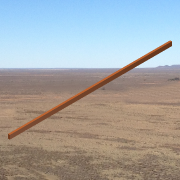
# Autodesk Inventor part: 2p4rim
Saved by Autodesk Inventor 2014 SP1 (Build 180222100, 222)
## iProperties
Company: HERA Project
Created: 2013-12-03
Part Number: 2p4rim
Material: Wood (Cherry)
Document SubType Name: Modeling
Designer: David DeBoer
Mass: 5807.17 g
Surface Area: 8777.4 cm^2
Volume: 11614.3 cm^3
Density: 0.5 g/cm^3
Description: rim piece
Appearance: Cherry - Natural Low Gloss
Author: David DeBoer
Autodesk Inventor part; units mm, degrees
ref_plane "YZ Plane" through (0, 0, 0) normal (1, 0, 0) x (0, 1, 0)
ref_plane "XZ Plane" through (0, 0, 0) normal (0, 1, 0) x (-1, 0, 0)
ref_plane "XY Plane" through (0, 0, 0) normal (0, 0, 1) x (1, 0, 0)
sketch "Sketch1" plane through (0, 0, 0) normal (0, 0, 1) x (1, 0, 0)
  line L0 (0, 0) -> (38.1, 0)
  line L1 (38.1, 0) -> (38.1, 88.9)
  line L2 (38.1, 88.9) -> (0, 88.9)
  line L3 (0, 88.9) -> (0, 0)
  dimension "d0" = 38.1
  dimension "d1" = 88.9
  constraints: 8 end point, 2 parallel, 1 horizontal, 1 perpendicular
  measures "d0" distance of L0.start L0.end
  measures "d1" distance of L2.end L0.start
extrude "Extrusion1" add sketch "Sketch1" along normal blind 3502.025
sketch "Sketch2" plane through (38.1, 0, 0) normal (0, -1, 0) x (1, 0, 0)
  line L0 (0, 0) -> (0, 3502.025) projected
  line L1 (-38.1, 0) -> (-38.1, 3502.025) projected
  line L2 (-38.1, 1751.0125) -> (0, 1751.0125) construction
  circle A0 centre (-19.05, 1763.7125) radius 1.4111
  circle A1 centre (-19.05, 1738.3125) radius 1.4111
  dimension "d4" = 12.7
  dimension "d8" = 25.4
  constraints: 2 centre point, 2 end point, 2 midpoint, 1 vertical, 2 other
  measures "d4" distance from line of L2 A0.centre
  measures "d8" distance of A0.centre A1.centre
hole "Hole1" at (19.05, 0, 1763.7125) at (19.05, 0, 1738.3125) direction (0, 1, 0) diameter 6.35 depth 25.4 tip angle 118
body "Solid1"
